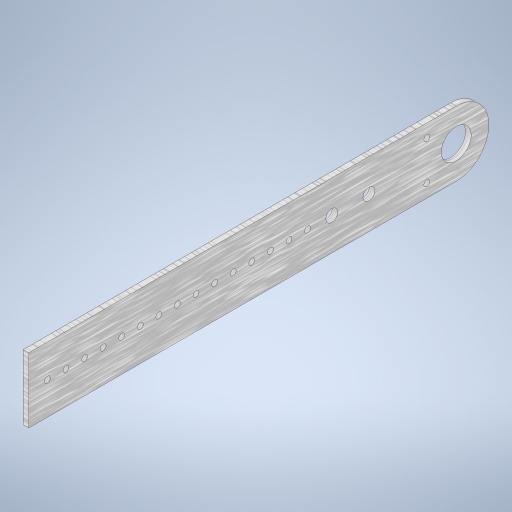
# Autodesk Inventor part: shoulder2_lower_left_plate
Saved by Autodesk Inventor 2024 (Build 280153000, 153)
## iProperties
Company: 細田研究室
Created: 2025-06-10
Part Number: shoulder2_lower_left_plate
Material: アルミニウム 5052
Document SubType Name: Modeling
Designer: HosodaLab2
Density: 2.68 g/cm^3
Appearance: サテン - ブラシ仕上げ 重厚
個数: 1
Author: HosodaLab2
Autodesk Inventor part; units mm, degrees
ref_plane "YZ Plane" through (0, 0, 0) normal (1, 0, 0) x (0, 1, 0)
ref_plane "XZ Plane" through (0, 0, 0) normal (0, 1, 0) x (-1, 0, 0)
ref_plane "XY Plane" through (0, 0, 0) normal (0, 0, 1) x (1, 0, 0)
sketch "スケッチ1" plane through (0, 0, 0) normal (0, 1, 0) x (-1, 0, 0)
  line L0 (0, 0) -> (-230, 0)
  line L1 (-230, 0) -> (-230, -35)
  line L2 (-230, -35) -> (0, -35)
  line L3 (0, -35) -> (0, 0)
  arc A0 (0, -35) -> (0, 0) centre (0, -17.5) ccw
  dimension "d0" = 230
  dimension "d1" = 35
  dimension "d2" = 17.5
  constraints: 8 end point, 2 parallel, 2 point on circle, 1 centre point, 1 horizontal, 1 perpendicular
  measures "d0" distance of L2.end L1.end
  measures "d1" distance of L1.end L0.end
  measures "d2" radius of A0
extrude "押し出し1" add sketch "スケッチ1" along normal blind 3
sketch "スケッチ2" plane through (0, 3, 0) normal (0, 1, 0) x (1, 0, 0)
  line L0 (0, 17.5) -> (238.6526, 17.5)
  line L1 (0, 0) -> (230, 0) projected
  arc A0 (0, 35) -> (0, 0) centre (0, 17.5) ccw projected
  point P0 (90, 17.5)
  point P1 (100, 17.5)
  point P2 (110, 17.5)
  point P3 (120, 17.5)
  point P4 (130, 17.5)
  point P5 (140, 17.5)
  point P6 (150, 17.5)
  point P7 (160, 17.5)
  point P8 (170, 17.5)
  point P9 (180, 17.5)
  point P10 (190, 17.5)
  point P11 (200, 17.5)
  point P12 (210, 17.5)
  point P13 (-17.5, 17.5)
  point P14 (220, 17.5)
  point P15 (80, 17.5)
  dimension "d5" = 17.5
  dimension "d13" = 10
  dimension "d14" = 10
  dimension "d15" = 10
  dimension "d16" = 10
  dimension "d17" = 10
  dimension "d18" = 10
  dimension "d19" = 10
  dimension "d20" = 10
  dimension "d21" = 10
  dimension "d22" = 10
  dimension "d23" = 10
  dimension "d24" = 10
  dimension "d35" = 17.5
  dimension "d67" = 10
  dimension "d78" = 10
  dimension "d96" = 80
  constraints: 1 point on circle, 18 other
  measures "d13" distance of point (100, 17.5) point (90, 17.5)
  measures "d14" distance of point (110, 17.5) point (100, 17.5)
  measures "d15" distance of point (120, 17.5) point (110, 17.5)
  measures "d16" distance of point (130, 17.5) point (120, 17.5)
  measures "d17" distance of point (140, 17.5) point (130, 17.5)
  measures "d18" distance of point (150, 17.5) point (140, 17.5)
  measures "d19" distance of point (160, 17.5) point (150, 17.5)
  measures "d20" distance of point (170, 17.5) point (160, 17.5)
  measures "d21" distance of point (180, 17.5) point (170, 17.5)
  measures "d22" distance of point (190, 17.5) point (180, 17.5)
  measures "d23" distance of point (200, 17.5) point (190, 17.5)
  measures "d24" distance of point (210, 17.5) point (200, 17.5)
  measures "d35" distance of point (-17.5, 17.5) point (0, 17.5)
  measures "d67" distance of point (210, 17.5) point (220, 17.5)
  measures "d78" distance of point (80, 17.5) point (90, 17.5)
  measures "d96" distance of point (80, 17.5) point (0, 17.5)
hole "穴1" at (90, 3, -17.5) at (100, 3, -17.5) at (110, 3, -17.5) at (120, 3, -17.5) at (130, 3, -17.5) at (140, 3, -17.5) at (150, 3, -17.5) at (160, 3, -17.5) at (170, 3, -17.5) at (180, 3, -17.5) at (190, 3, -17.5) at (200, 3, -17.5) at (210, 3, -17.5) at (220, 3, -17.5) at (80, 3, -17.5) direction (0, -1, 0) diameter 3.2 end through all
sketch "スケッチ3" plane through (0, 3, 0) normal (0, 1, 0) x (1, 0, 0)
  line L0 (230, 35) -> (0, 35) projected
  point P0 (0, 0)
  point P1 (0, 17.5)
  dimension "d36" = 17.5
  measures "d36" distance from line of L0 point (0, 17.5)
hole "穴2" at (0, 3, -17.5) direction (0, -1, 0) diameter 16 end through all
sketch "スケッチ4" plane through (0, 3, 0) normal (0, 1, 0) x (1, 0, 0)
  circle A0 centre (0, 17.5) radius 6
  circle A1 centre (0, 17.5) radius 8 projected
  line L0 (-0.1439, 17.5) -> (-6.5454, 17.5)
  line L1 (-6.5454, 17.5) -> (7.5104, 17.5)
  point P0 (0, 0)
  point P1 (0, 11.5)
  point P2 (6, 17.5)
  point P3 (0, 23.5)
  point P4 (-6, 17.5)
  dimension "d44" = 12
  dimension "d45" = 0
  constraints: 4 end point, 4 point on circle, 3 point on line, 1 centre point, 1 horizontal
  measures "d44" diameter of A0
  measures "d45" distance of A0.centre A1.centre
hole "穴3" [suppressed]
sketch "スケッチ5" plane through (0, 3, 0) normal (0, 1, 0) x (1, 0, 0)
  circle A0 centre (0, 17.5) radius 8 projected
  point P0 (0, 0)
  point P1 (15.8, 7)
  point P2 (15.8, 28)
  point P3 (24.9999, 17.5)
  dimension "d53" = 10.5
  dimension "d55" = 15.8
  dimension "d56" = 15.8
  dimension "d83" = 10.5
  measures "d53" vertical distance of point (25, 17.5) point (15.8, 7)
  measures "d55" horizontal distance of point (15.8, 7) A0.centre
  measures "d56" horizontal distance of A0.centre point (15.8, 28)
  measures "d83" vertical distance of point (15.8, 28) point (25, 17.5)
hole "穴4" at (15.8, 3, -28) at (15.8, 3, -7) direction (0, -1, 0) diameter 3.2 end through all
sketch "スケッチ6" plane through (0, 3, 0) normal (0, 1, 0) x (1, 0, 0)
  circle A0 centre (0, 17.5) radius 8 construction
  line L0 (0, 17.5) -> (230, 17.5) construction
  line L1 (230, 0) -> (230, 35) construction
  point P0 (0, 0)
  point P1 (67, 17.5)
  point P2 (47, 17.5)
  dimension "d69" = 47
  dimension "d70" = 20
  constraints: 2 end point, 2 point on line, 1 midpoint
  measures "d69" distance of point (47, 17.5) L0.start
  measures "d70" distance of point (67, 17.5) point (47, 17.5)
hole "穴5" at (67, 3, -17.5) at (47, 3, -17.5) direction (0, -1, 0) diameter 6.4 end through all
sketch "スケッチ7" plane through (0, 3, 0) normal (0, 1, 0) x (1, 0, 0)
  circle A0 centre (0, 17.5) radius 8 construction
  circle A1 centre (0, 17.5) radius 12.5 construction
  point P0 (0, 0)
  point P1 (0, 5)
  point P2 (12.5, 17.5)
  point P3 (0, 30)
  point P4 (-12.5, 17.5)
  dimension "d84" = 25
  dimension "d87" = 360
  constraints: 1 coincident, 1 vertical alignment, 7 other
hole "穴6" [suppressed]
